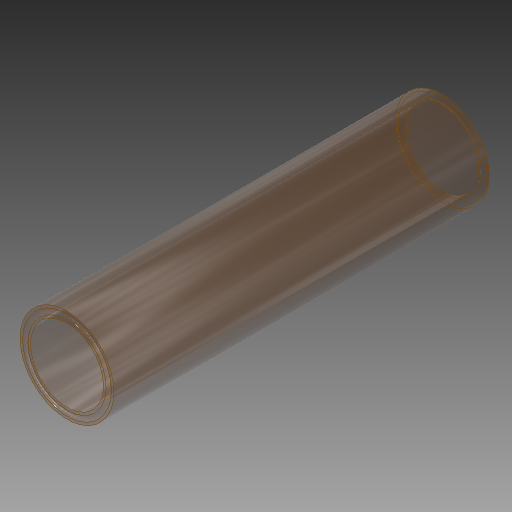
# Autodesk Inventor part: tube
Saved by Autodesk Inventor 2018.1 (Build 221171000, 171)
## iProperties
Created: 2017-08-10
Part Number: tube
Material: Polycarbonate, Smoke
Document SubType Name: Modeling
Designer: Kai
Density: 1.2 g/cm^3
Appearance: Polycarbonate - Smoked
Author: Kai
Autodesk Inventor part; units mm, degrees
ref_plane "YZ Plane" through (0, 0, 0) normal (1, 0, 0) x (0, 1, 0)
ref_plane "XZ Plane" through (0, 0, 0) normal (0, 1, 0) x (-1, 0, 0)
sketch "Sketch1" plane through (0, 0, 0) normal (0, 0, 1) x (1, 0, 0)
  circle A0 centre (0, 0) radius 22.225
  circle A1 centre (0, 0) radius 28.575
  dimension "d0" = 44.45
  dimension "d1" = 57.15
  constraints: 2 centre point, 2 coincident
  measures "d0" diameter of A0
  measures "d1" diameter of A1
extrude "Extrusion1" add sketch "Sketch1" along normal blind 228.6
sketch "Sketch2" plane through (0, 0, 228.6) normal (0, 0, 1) x (1, 0, 0)
  circle A0 centre (0, 0) radius 28.575 construction
  line L0 (0, 28.575) -> (0, -28.575) construction
  constraints: 2 end point, 2 point on circle, 1 vertical
ref_plane "Work Plane2" through (0, 0, 228.6) normal (0, 1, 0) x (-1, 0, 0)
ref_plane "Work Plane1" through (0, 28.575, 228.6) normal (0, 1, 0) x (-1, 0, 0)
sketch "Sketch3" plane through (0, 0, 228.6) normal (0, 1, 0) x (-1, 0, 0)
  line L0 (28.575, 0) -> (-28.575, 0) projected
  circle A0 centre (25.4, 0) radius 1.5875
  line L1 (0, 0) -> (0, 6.0913)
  line L2 (-28.575, -228.6) -> (28.575, -228.6) projected
  circle A1 centre (25.4, -228.6) radius 1.5875
  point P0 (0, -228.6)
  dimension "d5" = 3.175
  dimension "d6" = 25.4
  dimension "d7" = 3.175
  constraints: 2 centre point, 2 end point, 2 point on line, 1 midpoint, 1 vertical
  measures "d5" diameter of A0
  measures "d6" distance from line of L1 A0.centre
  measures "d7" diameter of A1
revolve "Revolution1" cut sketch "Sketch3" angle 360 about axis through (0, 0, 228.6) along (0, 0, 1)
body "Solid1"
